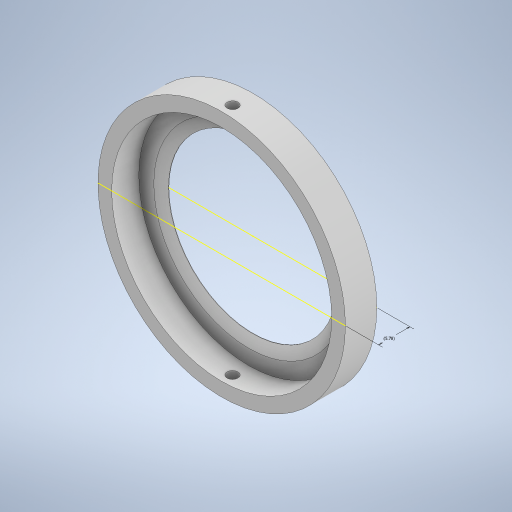
# Autodesk Inventor part: Diaphragm_lock
Saved by Autodesk Inventor 2023 (Build 270158000, 158)
## iProperties
Created: 2023-02-27
Part Number: Diaphragm_lock
Material: Generic
Document SubType Name: Modeling
Designer: maste
Density: 1 g/cm^3
Appearance: Default
Author: maste
Autodesk Inventor part; units mm, degrees
ref_plane "YZ Plane" through (0, 0, 0) normal (1, 0, 0) x (0, 1, 0)
ref_plane "XZ Plane" through (0, 0, 0) normal (0, 1, 0) x (-1, 0, 0)
ref_plane "XY Plane" through (0, 0, 0) normal (0, 0, 1) x (1, 0, 0)
sketch "Sketch1" plane through (0, 0, 0) normal (0, 0, 1) x (1, 0, 0)
  circle A0 centre (0, 0) radius 22.775
  dimension "d0" = 45.55
  constraints: 1 centre point, 1 coincident
  measures "d0" diameter of A0
extrude "Extrusion1" add sketch "Sketch1" along normal blind 5.78
sketch "Sketch2" plane through (0, 0, 5.78) normal (0, 0, 1) x (1, 0, 0)
  circle A0 centre (0, 0) radius 15.5
  dimension "d3" = 31
  constraints: 1 centre point, 1 coincident
  measures "d3" diameter of A0
extrude "Through-hole" cut sketch "Sketch2" against normal blind 548
sketch "Sketch3" plane through (0, 0, 5.78) normal (0, 0, 1) x (1, 0, 0)
  circle A0 centre (0, 0) radius 20.25
  dimension "d6" = 40.5
  constraints: 1 centre point, 1 coincident
  measures "d6" diameter of A0
extrude "snug ring fit" cut sketch "Sketch3" against normal blind 5
sketch "Sketch4" plane through (0, 0, 0) normal (0, 1, 0) x (-1, 0, 0)
  line L0 (22.775, 5.78) -> (-22.775, 5.78) projected
  line L1 (0, 5.78) -> (0, 3.78)
  circle A0 centre (0, 3.78) radius 1
  point P0 (0, 0)
  dimension "d9" = 2
  dimension "d10" = 2
  constraints: 2 end point, 1 centre point, 1 coincident, 1 midpoint, 1 vertical
  measures "d9" distance of L1.start L1.end
  measures "d10" diameter of A0
extrude "Extrusion4" cut sketch "Sketch4" along normal mid plane 548
chamfer "Chamfer1" distance 0.7 distance2 2 1 edges at (-15.5, 0, 0.78) measured on face at (-15.5, 0, 0.28)
sketch "Sketch5" plane through (0, 0, 0) normal (0, 1, 0) x (-1, 0, 0)
  line L0 (22.775, 5.78) -> (-22.775, 5.78) projected
  line L1 (22.775, 0) -> (-22.775, 0) projected
  point P0 (0, 0)
  dimension "d16" = 5.78
  measures "d16" distance between parallel lines of L0 L1
body "Solid1"
